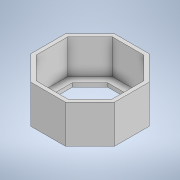
# Autodesk Inventor part: TokenHolderSingle
Saved by Autodesk Inventor 2020 (Build 240168000, 168)
## iProperties
Created: 2020-06-16
Part Number: TokenHolderSingle
Material: Generic
Document SubType Name: Modeling
Designer: user
Density: 1 g/cm^3
Appearance: Default
Author: user
## iProperties of the stored document _3DPrint.ipt
Created: 2020-06-18
Part Number: _3DPrint
Material: Generic
Document SubType Name: Modeling
Designer: user
Density: 1 g/cm^3
Appearance: Default
Author: user
Autodesk Inventor part; units mm, degrees
ref_plane "YZ Plane" through (0, 0, 0) normal (1, 0, 0) x (0, 1, 0)
ref_plane "XZ Plane" through (0, 0, 0) normal (0, 1, 0) x (-1, 0, 0)
ref_plane "XY Plane" through (0, 0, 0) normal (0, 0, 1) x (1, 0, 0)
sketch "Sketch1" plane through (0, 0, 0) normal (0, 1, 0) x (-1, 0, 0)
  line L0 (7.5264, 21.8341) -> (7.5264, 13.5841)
  line L1 (7.5264, 13.5841) -> (1.6928, 7.7505)
  line L2 (1.6928, 7.7505) -> (-6.5572, 7.7505)
  line L3 (7.5264, 21.8341) -> (1.6928, 27.6678)
  line L4 (1.6928, 27.6678) -> (-6.5572, 27.6678)
  line L5 (-6.5572, 27.6678) -> (-12.3908, 21.8341)
  line L6 (-12.3908, 21.8341) -> (-12.3908, 13.5841)
  line L7 (-12.3908, 13.5841) -> (-6.5572, 7.7505)
  line L8 (8.5264, 22.2483) -> (8.5264, 13.1699)
  line L9 (8.5264, 13.1699) -> (2.107, 6.7505)
  line L10 (2.107, 6.7505) -> (-6.9714, 6.7505)
  line L11 (8.5264, 22.2483) -> (2.107, 28.6678)
  line L12 (2.107, 28.6678) -> (-6.9714, 28.6678)
  line L13 (-6.9714, 28.6678) -> (-13.3908, 22.2483)
  line L14 (-13.3908, 22.2483) -> (-13.3908, 13.1699)
  line L15 (-13.3908, 13.1699) -> (-6.9714, 6.7505)
  point P0 (0, 0)
  point P1 (1, 1)
  dimension "d0" = 8.25
  dimension "d3" = 8.25
  dimension "d5" = 8.25
  dimension "d7" = 8.25
  dimension "d8" = 8.25
  dimension "d9" = 8.25
  dimension "d12" = 8.25
  dimension "d17" = 8.25
  dimension "d29" = 1
  dimension "d31" = 1
  dimension "d32" = 1
  dimension "d33" = 1
  dimension "d101" = 135
  dimension "d102" = 135
  dimension "d115" = 135
  dimension "d116" = 135
  dimension "d135" = 1
  dimension "d138" = 1
  dimension "d139" = 135
  dimension "d140" = 135
  dimension "d141" = 135
  dimension "d142" = 135
  dimension "d143" = 1
  dimension "d144" = 1
  dimension "d145" = 135
  dimension "d146" = 135
  dimension "d147" = 135
  dimension "d148" = 135
  dimension "d149" = 135
  dimension "d150" = 135
  dimension "d151" = 135
  dimension "d152" = 135
  constraints: 32 end point, 4 horizontal, 4 vertical
  measures "d0" distance of L0.end L0.start
  measures "d3" distance of L0.end L1.end
  measures "d5" distance of L1.end L2.end
  measures "d7" distance of L0.start L3.end
  measures "d8" distance of L3.end L4.end
  measures "d9" distance of L4.end L5.end
  measures "d12" distance of L5.end L6.end
  measures "d17" distance of L6.end L2.end
  measures "d29" distance between parallel lines of L14 L6
  measures "d31" distance between parallel lines of L12 L4
  measures "d32" distance between parallel lines of L10 L2
  measures "d33" distance between parallel lines of L0 L8
  measures "d101" angle of L0 L1
  measures "d102" angle of L1 L2
  measures "d115" angle of L9 L10
  measures "d116" angle of L8 L9
  measures "d135" distance between parallel lines of L1 L9
  measures "d138" distance between parallel lines of L15 L7
  measures "d139" angle of L7 L2
  measures "d140" angle of L15 L10
  measures "d141" angle of L14 L15
  measures "d142" angle of L6 L7
  measures "d143" distance between parallel lines of L13 L5
  measures "d144" distance between parallel lines of L11 L3
  measures "d145" angle of L3 L0
  measures "d146" angle of L4 L3
  measures "d147" angle of L5 L4
  measures "d148" angle of L5 L6
  measures "d149" angle of L11 L8
  measures "d150" angle of L12 L11
  measures "d151" angle of L13 L12
  measures "d152" angle of L14 L13
extrude "OutsideHeight" add sketch "Sketch1" along normal blind 10
extrude "BaseHeight" add sketch "Sketch1" along normal blind 1 contours L0 L1 L2 L7 L6 L5 L4 L3
sketch "Sketch5" plane through (0, 1, 0) normal (0, 1, 0) x (1, 0, 0)
  line L0 (-1.6928, -27.6678) -> (-7.5264, -21.8341) projected
  line L1 (-7.5264, -13.5841) -> (-1.6928, -7.7505) projected
  line L2 (-7.5264, -21.8341) -> (-7.5264, -13.5841)
  line L3 (-7.5264, -13.5841) -> (-1.6928, -7.7505)
  line L4 (-1.6928, -7.7505) -> (6.5572, -7.7505) projected
  line L5 (-1.6928, -7.7505) -> (6.5572, -7.7505)
  line L6 (6.5572, -7.7505) -> (12.3908, -13.5841)
  line L7 (12.3908, -13.5841) -> (12.7122, -18.5063)
  line L8 (12.3908, -13.5841) -> (12.3908, -21.8341) projected
  line L9 (12.3908, -13.5841) -> (12.3908, -21.8341)
  line L10 (12.3908, -21.8341) -> (6.5572, -27.6678)
  line L11 (6.5572, -27.6678) -> (-1.6928, -27.6678)
  line L12 (-1.6928, -27.6678) -> (-7.5264, -21.8341)
  line L13 (-5.5264, -21.0057) -> (-5.5264, -14.4125)
  line L14 (-5.5264, -14.4125) -> (-0.8644, -9.7505)
  line L15 (-0.8644, -9.7505) -> (5.7288, -9.7505)
  line L16 (5.7288, -9.7505) -> (10.3908, -14.4125)
  line L17 (10.3908, -14.4125) -> (10.3908, -21.0057)
  line L18 (10.3908, -21.0057) -> (5.7288, -25.6678)
  line L19 (5.7288, -25.6678) -> (-0.8644, -25.6678)
  line L20 (-0.8644, -25.6678) -> (-5.5264, -21.0057)
  point P0 (0, 0)
  point P1 (-1.6932, -27.6674)
  dimension "d94" = 135
  dimension "d95" = 135
  dimension "d125" = 135
  dimension "d126" = 135
  dimension "d127" = 135
  dimension "d128" = 135
  dimension "d129" = 135
  dimension "d130" = 135
  dimension "d131" = 2
  constraints: 34 end point, 3 collinear, 2 perpendicular, 1 vertical, 7 other
  measures "d94" angle of L4 L6
  measures "d95" angle of L4 L1
  measures "d125" angle of L2 L12
  measures "d126" angle of L1 L2
  measures "d127" angle of L12 L11
  measures "d128" angle of L10 L11
  measures "d129" angle of L8 L10
  measures "d130" angle of L6 L8
  measures "d131" distance between parallel lines of L12 L20
extrude "BaseCut" cut sketch "Sketch5" against normal blind 1 contours L13 L14 L15 L16 L17 L18 L19 L20
equation "\"d3\" = d0"
equation "\"d5\" = d0"
equation "\"d7\" = d0"
equation "\"d8\" = d0"
equation "\"d9\" = d0"
equation "\"d12\" = d0"
equation "\"d17\" = d0"
equation "\"d115\" = d110"
equation "\"d57\" = d72"
equation "\"d66\" = d57"
equation "\"d110\" = 135deg"
equation "\"d72\" = 2"
body "Solid1"
